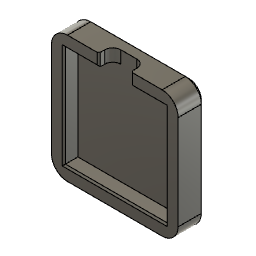
LED_mount_brick (Autodesk Fusion 360 design; units mm, degrees)
Autodesk Fusion 360 part; units mm, degrees
sketch "Sketch1" plane through (0, 0, 0) normal (0, 0, 1) x (1, 0, 0)
  line L0 (-7.9, 7.9) -> (7.9, 7.9)
  line L1 (7.9, 7.9) -> (7.9, -7.9)
  line L2 (7.9, -7.9) -> (-7.9, -7.9)
  line L3 (-7.9, -7.9) -> (-7.9, 7.9)
  line L4 (-7.9, 7.9) -> (7.9, -7.9) construction
  line L5 (7.9, 7.9) -> (-7.9, -7.9) construction
  dimension "d1" = 15.8
  constraint horizontal L0
  constraint perpendicular L0 L1
  constraint parallel L0 L2
  constraint parallel L1 L3
  constraint coincident L4 origin
  constraint coincident L5 origin
  constraint equal L0 L1
  measures "d1" distance of L0.end L1.end
extrude "Extrude1" add sketch "Sketch1" along normal blind 3.3
shell "Shell1" thickness 1.55 removed faces 1 at (-2.6333, 2.6333, 3.3)
fillet "Fillet1" radius 2 4 edges at (7.9, 7.9, 1.65) (7.9, -7.9, 1.65) (-7.9, -7.9, 1.65) (-7.9, 7.9, 1.65)
chamfer "Chamfer1" distance 0.4 angle 45 8 edges at (7.9, 0, 0) (7.3142, -7.3142, 0) (0, -7.9, 0) (-7.3142, -7.3142, 0) (-7.9, 0, 0) (-7.3142, 7.3142, 0) (0, 7.9, 0) (7.3142, 7.3142, 0)
chamfer "Chamfer2" distance 0.2 angle 45 4 edges at (-6.35, 0, 3.3) (0, 6.35, 3.3) (6.35, 0, 3.3) (0, -6.35, 3.3)
sketch "Sketch2" plane through (0, 0, 3.3) normal (0, 0, 1) x (1, 0, 0)
  arc A0 (-5.9, 7.9) -> (-7.9, 5.9) centre (-5.9, 5.9) ccw
  line L0 (-7.9, 5.9) -> (-7.9, -5.9)
  arc A1 (-7.9, -5.9) -> (-5.9, -7.9) centre (-5.9, -5.9) ccw
  line L1 (-5.9, -7.9) -> (5.9, -7.9)
  arc A2 (5.9, -7.9) -> (7.9, -5.9) centre (5.9, -5.9) ccw
  line L2 (7.9, -5.9) -> (7.9, 5.9)
  arc A3 (7.9, 5.9) -> (5.9, 7.9) centre (5.9, 5.9) ccw
  line L3 (5.9, 7.9) -> (-5.9, 7.9)
  line L4 (-6.55, -6.55) -> (-6.55, 6.55)
  line L5 (-6.55, 6.55) -> (6.55, 6.55)
  line L6 (6.55, 6.55) -> (6.55, -6.55)
  line L7 (6.55, -6.55) -> (-6.55, -6.55)
  line L8 (0, 0) -> (0, 7.9) construction
  line L9 (2, 6.0755) -> (-2, 6.0755)
  line L10 (-2, 6.0755) -> (-2, 9.7245)
  line L11 (-2, 9.7245) -> (2, 9.7245)
  line L12 (2, 9.7245) -> (2, 6.0755)
  line L13 (2, 6.0755) -> (-2, 9.7245) construction
  line L14 (-2, 6.0755) -> (2, 9.7245) construction
  point P0 (0, 7.9)
  dimension "d9" = 4
  constraint coincident L8.start origin
  constraint midpoint L3 P0
  constraint horizontal L9
  constraint perpendicular L9 L10
  constraint parallel L9 L11
  constraint parallel L10 L12
  constraint coincident L13 P0
  constraint coincident L14 P0
  constraint coincident P0 L8.end
  measures "d9" distance of L10.end L11.end
extrude "Extrude2" cut sketch "Sketch2" against normal up to surface (1.75 mm away) contours L3 L10 L11 L12 | L3 L5 L10 L12 | L5 L9 L10 L12
fillet "Fillet2" radius 1 2 edges at (-2, 7.125, 1.55) (2, 7.125, 1.55)
chamfer "Chamfer3" distance 0.2 angle 45 2 edges at (2, 7.225, 3.3) (-2, 7.225, 3.3)
